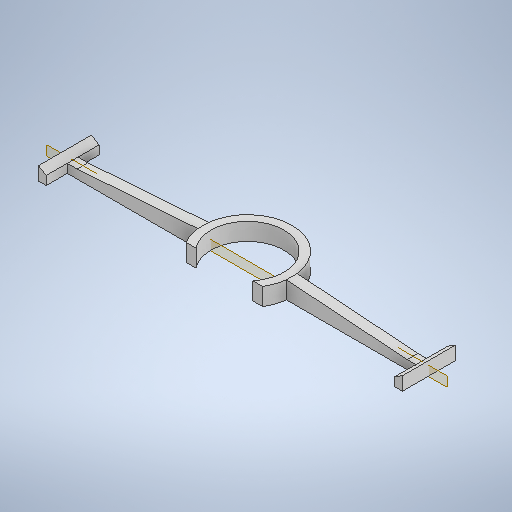
# Autodesk Inventor part: 2024_08_28_Holder_GL25
Saved by Autodesk Inventor 2025.1 (Build 291241000, 241)
## iProperties
Created: 2024-08-23
Part Number: 2024_08_28_Holder_GL25
Material: Generisch
Document SubType Name: Modeling
Designer: to86hug
Density: 1 g/cm^3
Appearance: Vorgabe
Author: to86hug
Autodesk Inventor part; units mm, degrees
ref_plane "YZ Plane" through (0, 0, 0) normal (1, 0, 0) x (0, 1, 0)
ref_plane "XZ Plane" through (0, 0, 0) normal (0, 1, 0) x (-1, 0, 0)
ref_plane "XY Plane" through (0, 0, 0) normal (0, 0, 1) x (1, 0, 0)
sketch "Skizze1" plane through (0, 0, 0) normal (0, 0, 1) x (1, 0, 0)
  line L0 (-68.016, 1.808) -> (67.584, 1.808)
  line L1 (67.584, 1.808) -> (67.584, -2.192)
  line L2 (67.584, -2.192) -> (-68.016, -2.192)
  line L3 (-68.016, -2.192) -> (-68.016, 1.808)
  line L4 (-68.016, 1.808) -> (67.584, -2.192) construction
  line L5 (67.584, 1.808) -> (-68.016, -2.192) construction
  point P0 (0, 0)
  point P1 (-0.216, -0.192)
  point P2 (-0.216, -0.192)
  dimension "d0" = 135.6
  dimension "d1" = 4
  constraints: 12 end point, 2 midpoint, 2 parallel, 1 horizontal, 1 perpendicular
  measures "d0" distance of L0.start L0.end
  measures "d1" distance of L0.end L1.end
extrude "Extrusion1" add sketch "Skizze1" along normal mid plane 3.25
ref_plane "Arbeitsebene1" through (-68.016, -0.192, 1.625) normal (0, -1, 0) x (1, 0, 0)
sketch "Skizze2" plane through (-68.016, -0.192, 1.625) normal (0, -1, 0) x (1, 0, 0)
  line L0 (0, -3.25) -> (0, 0) projected
  line L1 (0, -3.25) -> (135.6, -3.25) projected
  line L2 (0, 0) -> (2.85, 0)
  line L3 (2.85, 0) -> (2.85, -3.25)
  line L4 (2.85, -3.25) -> (0, -3.25)
  line L5 (0, -3.25) -> (0, 0)
  line L6 (0, 0) -> (0, 1.75)
  line L7 (0, 1.75) -> (2.85, 0)
  line L8 (135.6, -3.25) -> (135.6, 0) projected
  line L9 (135.6, 0) -> (132.75, 0)
  line L10 (132.75, 0) -> (132.75, -3.25)
  line L11 (132.75, -3.25) -> (135.6, -3.25)
  line L12 (135.6, -3.25) -> (135.6, 0)
  line L13 (135.6, 0) -> (135.6, 1.75)
  line L14 (135.6, 1.75) -> (132.75, 0)
  point P0 (68.016, -1.625)
  dimension "d4" = 2.85
  dimension "d5" = 1.75
  dimension "d6" = 2.85
  constraints: 24 end point, 4 parallel, 2 horizontal, 2 perpendicular, 2 point on line, 2 vertical
  measures "d4" distance of L3.end L4.end
  measures "d5" distance of L0.end L6.end
  measures "d6" distance of L11.end L10.end
extrude "Extrusion2" add sketch "Skizze2" along normal mid plane 19.7
sketch "Skizze3" plane through (0, 0, 1.625) normal (0, 0, 1) x (1, 0, 0)
  circle A0 centre (0, 0) radius 16
  dimension "d9" = 32
  constraints: 1 centre point, 1 coincident
  measures "d9" diameter of A0
extrude "Extrusion3" cut sketch "Skizze3" against normal through all
sketch "Skizze4" plane through (0, 0, -1.625) normal (0, 0, -1) x (-1, 0, 0)
  line L0 (0.0777, -0.1628) -> (6.2277, -0.1628) construction
  circle A0 centre (0.0009, -0.1935) radius 13.625
  circle A1 centre (0.0009, -0.1935) radius 16.625
  line L1 (-22.383, -8.7935) -> (26.817, -8.7935)
  point P0 (-16.6241, -0.1935)
  point P1 (16.6259, -0.1935)
  point P2 (10.5688, -8.7935)
  point P3 (14.2287, -8.7935)
  point P4 (-14.2269, -8.7935)
  point P5 (-10.567, -8.7935)
  dimension "d27" = 3
  dimension "d28" = 27.25
  dimension "d29" = 8.6
  constraints: 4 end point, 2 centre point, 2 coincident, 2 point on circle
  measures "d27" radial gap between concentric circles of A1 A0
  measures "d28" diameter of A0
  measures "d29" distance from line of A0.centre L1
extrude "Extrusion4" add sketch "Skizze4" against normal blind 6.5 contours A0 L1 A1 picked at (15.3303, 2.2297)
sketch "Skizze7" plane through (0, 0, 1.625) normal (0, 0, 1) x (1, 0, 0)
  line L0 (-65.166, 1.808) -> (-16.5049, 1.808) projected
  line L1 (-16.5053, -2.192) -> (-65.166, -2.192) projected
  line L2 (-16.5049, 1.808) -> (-61.5049, 1.808)
  line L3 (-61.5049, 1.808) -> (-61.5049, -2.192)
  line L4 (-61.5049, -2.192) -> (-16.5049, -2.192)
  line L5 (-16.5049, -2.192) -> (-16.5049, 1.808)
  line L6 (16.5032, 1.808) -> (64.734, 1.808) projected
  line L7 (64.734, -2.192) -> (16.5036, -2.192) projected
  line L8 (16.5032, 1.808) -> (61.5032, 1.808)
  line L9 (61.5032, 1.808) -> (61.5032, -2.192)
  line L10 (61.5032, -2.192) -> (16.5032, -2.192)
  line L11 (16.5032, -2.192) -> (16.5032, 1.808)
  point P0 (0, 0)
  point P1 (-61.5049, 1.808)
  point P2 (16.5036, -2.192)
  point P3 (61.5032, 1.808)
  dimension "d30" = 45
  dimension "d31" = 45
  constraints: 16 end point, 4 parallel, 2 horizontal, 2 perpendicular, 2 point on line
  measures "d30" distance of L4.end L3.end
  measures "d31" distance of L9.end L10.end
extrude "Extrusion7" add sketch "Skizze7" along normal blind 3.25
sketch "Skizze8" plane through (-65.166, -2.192, -1.625) normal (0, -1, 0) x (1, 0, 0)
  line L0 (48.661, 6.5) -> (3.661, 6.5) projected
  line L1 (48.661, 6.5) -> (48.661, 0) projected
  line L2 (3.661, 6.5) -> (48.661, 6.5)
  line L3 (48.661, 6.5) -> (48.661, 3.25)
  line L4 (48.661, 3.25) -> (3.661, 3.25)
  line L5 (3.661, 3.25) -> (3.661, 6.5)
  line L6 (126.6692, 3.25) -> (126.6692, 6.5) projected
  line L7 (81.6692, 6.5) -> (81.6692, 0) projected
  line L8 (126.6692, 6.5) -> (81.6692, 6.5)
  line L9 (81.6692, 6.5) -> (81.6692, 3.25)
  line L10 (81.6692, 3.25) -> (126.6692, 3.25)
  line L11 (126.6692, 3.25) -> (126.6692, 6.5)
  line L12 (81.6692, 6.5) -> (126.6692, 3.25)
  line L13 (50.9373, 6.5) -> (48.6607, 6.5) projected
  line L14 (48.6607, 6.5) -> (3.661, 3.25)
  point P0 (65.166, 1.625)
  constraints: 20 end point, 4 parallel, 2 horizontal, 2 midpoint, 2 perpendicular
extrude "Extrusion8" cut sketch "Skizze8" against normal through all contours L14 L5 L0 | L12 L8 L6
